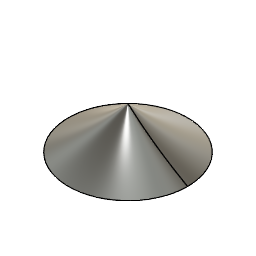
独自ミラー 試作品1 (Autodesk Fusion 360 design; units mm, degrees)
Autodesk Fusion 360 part; units mm, degrees
sketch "スケッチ2" plane through (0, 0, 0) normal (0, 0, 1) x (1, 0, 0)
  spline S0 degree 5 poles (25.9808, 45) (25.9662, 44.9918) (25.9371, 44.9754) (25.8935, 44.9508) (25.8354, 44.918) (25.7629, 44.8771) (25.6905, 44.8361) (25.6181, 44.7952) (25.5459, 44.7542) (25.4738, 44.7133) (25.4017, 44.6724) (25.3298, 44.6316) (25.2579, 44.5907) (25.1862, 44.5499) (25.1145, 44.509) (25.0429, 44.4682) (24.9715, 44.4274) (24.9001, 44.3866) (24.8288, 44.3459) (24.7576, 44.3051) (24.6865, 44.2644) (24.6155, 44.2236) (24.5446, 44.1829) (24.4738, 44.1422) (24.403, 44.1016) (24.3324, 44.0609) (24.2619, 44.0203) (24.1914, 43.9796) (24.1211, 43.939) (24.0508, 43.8984) (23.9806, 43.8578) (23.9106, 43.8172) (23.8406, 43.7767) (23.7707, 43.7361) (23.7009, 43.6956) (23.6312, 43.6551) (23.5616, 43.6146) (23.4921, 43.5741) (23.4227, 43.5336) (23.3533, 43.4932) (23.2841, 43.4528) (23.215, 43.4123) (23.1459, 43.3719) (23.0769, 43.3315) (23.0081, 43.2912) (22.9393, 43.2508) (22.8706, 43.2104) (22.802, 43.1701) (22.7335, 43.1298) (22.6651, 43.0895) (22.5968, 43.0492) (22.5286, 43.0089) (22.4604, 42.9687) (22.3924, 42.9284) (22.3244, 42.8882) (22.2566, 42.848) (22.1888, 42.8078) (22.1211, 42.7676) (22.0535, 42.7275) (21.986, 42.6873) (21.9186, 42.6472) (21.8513, 42.6071) (21.7841, 42.567) (21.717, 42.5269) (21.6499, 42.4868) (21.583, 42.4467) (21.5161, 42.4067) (21.4493, 42.3667) (21.3826, 42.3267) (21.316, 42.2867) (21.2495, 42.2467) (21.1831, 42.2067) (21.1168, 42.1668) (21.0506, 42.1268) (20.9844, 42.0869) (20.9184, 42.047) (20.8524, 42.0071) (20.7865, 41.9672) (20.7207, 41.9274) (20.655, 41.8875) (20.5894, 41.8477) (20.5239, 41.8079) (20.4585, 41.7681) (20.3931, 41.7283) (20.3279, 41.6885) (20.2627, 41.6488) (20.1976, 41.609) (20.1327, 41.5693) (20.0678, 41.5296) (20.0029, 41.4899) (19.9382, 41.4502) (19.8736, 41.4106) (19.809, 41.3709) (19.7446, 41.3313) (19.6802, 41.2917) (19.6159, 41.2521) (19.5517, 41.2125) (19.4876, 41.1729) (19.4236, 41.1334) (19.3597, 41.0938) (19.2959, 41.0543) (19.2321, 41.0148) (19.1684, 40.9753) (19.1049, 40.9358) (19.0414, 40.8963) (18.978, 40.8569) (18.9146, 40.8175) (18.8514, 40.778) (18.7883, 40.7386) (18.7252, 40.6993) (18.6622, 40.6599) (18.5993, 40.6205) (18.5365, 40.5812) (18.4738, 40.5419) (18.4112, 40.5025) (18.3487, 40.4632) (18.2862, 40.424) (18.2239, 40.3847) (18.1616, 40.3454) (18.0994, 40.3062) (18.0373, 40.267) (17.9753, 40.2278) (17.9133, 40.1886) (17.8515, 40.1494) (17.7897, 40.1103) (17.728, 40.0711) (17.6664, 40.032) (17.6049, 39.9929) (17.5435, 39.9538) (17.4822, 39.9147) (17.4209, 39.8756) (17.3597, 39.8366) (17.2987, 39.7976) (17.2377, 39.7585) (17.1768, 39.7195) (17.1159, 39.6805) (17.0552, 39.6416) (16.9945, 39.6026) (16.934, 39.5637) (16.8735, 39.5247) (16.8131, 39.4858) (16.7527, 39.4469) (16.6925, 39.408) (16.6324, 39.3692) (16.5723, 39.3303) (16.5123, 39.2915) (16.4524, 39.2527) (16.3926, 39.2139) (16.3329, 39.1751) (16.2732, 39.1363) (16.2136, 39.0975) (16.1542, 39.0588) (16.0948, 39.0201) (16.0355, 38.9814) (15.9762, 38.9427) (15.9171, 38.904) (15.858, 38.8653) (15.799, 38.8267) (15.7401, 38.788) (15.6813, 38.7494) (15.6226, 38.7108) (15.5639, 38.6722) (15.5054, 38.6336) (15.4469, 38.5951) (15.3885, 38.5565) (15.3302, 38.518) (15.2719, 38.4795) (15.2138, 38.441) (15.1557, 38.4025) (15.0977, 38.3641) (15.0398, 38.3256) (14.982, 38.2872) (14.9242, 38.2488) (14.8666, 38.2104) (14.809, 38.172) (14.7515, 38.1336) (14.6941, 38.0952) (14.6367, 38.0569) (14.5795, 38.0186) (14.5223, 37.9803) (14.4652, 37.942) (14.4082, 37.9037) (14.3513, 37.8654) (14.2944, 37.8272) (14.2377, 37.7889) (14.181, 37.7507) (14.1244, 37.7125) (14.0679, 37.6743) (14.0114, 37.6362) (13.955, 37.598) (13.8988, 37.5599) (13.8426, 37.5217) (13.7864, 37.4836) (13.7304, 37.4455) (13.6744, 37.4075) (13.6186, 37.3694) (13.5628, 37.3314) (13.507, 37.2933) (13.4514, 37.2553) (13.3958, 37.2173) (13.3403, 37.1793) (13.2849, 37.1414) (13.2296, 37.1034) (13.1744, 37.0655) (13.1192, 37.0276) (13.0641, 36.9897) (13.0091, 36.9518) (12.9542, 36.9139) (12.8994, 36.876) (12.8446, 36.8382) (12.7899, 36.8004) (12.7353, 36.7626) (12.6808, 36.7248) (12.6263, 36.687) (12.5719, 36.6492) (12.5176, 36.6115) (12.4634, 36.5737) (12.4093, 36.536) (12.3552, 36.4983) (12.3012, 36.4606) (12.2473, 36.423) (12.1935, 36.3853) (12.1398, 36.3477) (12.0861, 36.31) (12.0325, 36.2724) (11.979, 36.2349) (11.9256, 36.1973) (11.8722, 36.1597) (11.8189, 36.1222) (11.7657, 36.0846) (11.7126, 36.0471) (11.6595, 36.0096) (11.6066, 35.9722) (11.5537, 35.9347) (11.5009, 35.8972) (11.4481, 35.8598) (11.3955, 35.8224) (11.3429, 35.785) (11.2904, 35.7476) (11.2379, 35.7102) (11.1856, 35.6729) (11.1333, 35.6356) (11.0811, 35.5982) (11.029, 35.5609) (10.9769, 35.5236) (10.925, 35.4864) (10.8731, 35.4491) (10.8212, 35.4119) (10.7695, 35.3746) (10.7178, 35.3374) (10.6662, 35.3002) (10.6147, 35.2631) (10.5633, 35.2259) (10.5119, 35.1888) (10.4606, 35.1516) (10.4094, 35.1145) (10.3583, 35.0774) (10.3072, 35.0403) (10.2562, 35.0033) (10.2053, 34.9662) (10.1545, 34.9292) (10.1037, 34.8922) (10.053, 34.8552) (10.0024, 34.8182) (9.9519, 34.7812) (9.9014, 34.7443) (9.851, 34.7073) (9.8007, 34.6704) (9.7505, 34.6335) (9.7003, 34.5966) (9.6502, 34.5597) (9.6002, 34.5229) (9.5502, 34.4861) (9.5004, 34.4492) (9.4506, 34.4124) (9.4009, 34.3756) (9.3512, 34.3389) (9.3016, 34.3021) (9.2521, 34.2654) (9.2027, 34.2286) (9.1534, 34.1919) (9.1041, 34.1552) (9.0549, 34.1186) (9.0057, 34.0819) (8.9567, 34.0453) (8.9077, 34.0086) (8.8588, 33.972) (8.8099, 33.9354) (8.7612, 33.8989) (8.7125, 33.8623) (8.6639, 33.8258) (8.6153, 33.7892) (8.5668, 33.7527) (8.5184, 33.7162) (8.4701, 33.6797) (8.4218, 33.6433) (8.3737, 33.6068) (8.3255, 33.5704) (8.2775, 33.534) (8.2295, 33.4976) (8.1816, 33.4612) (8.1338, 33.4249) (8.0861, 33.3885) (8.0384, 33.3522) (7.9908, 33.3159) (7.9432, 33.2796) (7.8958, 33.2433) (7.8484, 33.2071) (7.801, 33.1708) (7.7538, 33.1346) (7.7066, 33.0984) (7.6595, 33.0622) (7.6124, 33.026) (7.5655, 32.9899) (7.5186, 32.9537) (7.4717, 32.9176) (7.425, 32.8815) (7.3783, 32.8454) (7.3317, 32.8093) (7.2851, 32.7733) (7.2387, 32.7372) (7.1923, 32.7012) (7.1459, 32.6652) (7.0997, 32.6292) (7.0535, 32.5933) (7.0073, 32.5573) (6.9613, 32.5214) (6.9153, 32.4855) (6.8694, 32.4496) (6.8235, 32.4137) (6.7778, 32.3778) (6.7321, 32.342) (6.6864, 32.3061) (6.6408, 32.2703) (6.5953, 32.2345) (6.5499, 32.1988) (6.5046, 32.163) (6.4593, 32.1273) (6.414, 32.0915) (6.3689, 32.0558) (6.3238, 32.0201) (6.2788, 31.9845) (6.2338, 31.9488) (6.189, 31.9132) (6.1441, 31.8776) (6.0994, 31.842) (6.0547, 31.8064) (6.0101, 31.7708) (5.9656, 31.7353) (5.9211, 31.6998) (5.8767, 31.6643) (5.8324, 31.6288) (5.7881, 31.5933) (5.7439, 31.5579) (5.6998, 31.5224) (5.6557, 31.487) (5.6117, 31.4516) (5.5678, 31.4163) (5.5239, 31.3809) (5.4801, 31.3456) (5.4364, 31.3103) (5.3927, 31.275) (5.3491, 31.2397) (5.3056, 31.2044) (5.2621, 31.1692) (5.2187, 31.1339) (5.1754, 31.0987) (5.1321, 31.0636) (5.0889, 31.0284) (5.0458, 30.9933) (5.0027, 30.9581) (4.9597, 30.923) (4.9168, 30.8879) (4.8739, 30.8529) (4.8311, 30.8178) (4.7884, 30.7828) (4.7457, 30.7478) (4.7031, 30.7128) (4.6606, 30.6778) (4.6181, 30.6429) (4.5757, 30.608) (4.5333, 30.5731) (4.491, 30.5382) (4.4488, 30.5033) (4.4067, 30.4685) (4.3646, 30.4337) (4.3226, 30.3989) (4.2806, 30.3641) (4.2387, 30.3293) (4.1969, 30.2946) (4.1551, 30.2599) (4.1134, 30.2252) (4.0718, 30.1905) (4.0302, 30.1559) (3.9887, 30.1213) (3.9472, 30.0867) (3.9058, 30.0521) (3.8645, 30.0175) (3.8232, 29.983) (3.782, 29.9485) (3.7409, 29.914) (3.6998, 29.8795) (3.6588, 29.8451) (3.6179, 29.8107) (3.577, 29.7763) (3.5362, 29.7419) (3.4954, 29.7076) (3.4547, 29.6732) (3.4141, 29.6389) (3.3735, 29.6047) (3.333, 29.5704) (3.2925, 29.5362) (3.2521, 29.502) (3.2118, 29.4678) (3.1715, 29.4337) (3.1313, 29.3996) (3.0912, 29.3655) (3.0511, 29.3314) (3.011, 29.2974) (2.9711, 29.2634) (2.9311, 29.2294) (2.8913, 29.1955) (2.8515, 29.1615) (2.8118, 29.1276) (2.7721, 29.0938) (2.7325, 29.0599) (2.6929, 29.0261) (2.6534, 28.9924) (2.614, 28.9586) (2.5746, 28.9249) (2.5353, 28.8912) (2.496, 28.8576) (2.4568, 28.824) (2.4177, 28.7904) (2.3786, 28.7568) (2.3395, 28.7233) (2.3006, 28.6898) (2.2616, 28.6564) (2.2228, 28.623) (2.1839, 28.5896) (2.1452, 28.5563) (2.1065, 28.523) (2.0678, 28.4897) (2.0292, 28.4565) (1.9907, 28.4234) (1.9522, 28.3902) (1.9138, 28.3571) (1.8754, 28.3241) (1.8371, 28.2911) (1.7988, 28.2581) (1.7606, 28.2252) (1.7224, 28.1924) (1.6843, 28.1596) (1.6462, 28.1268) (1.6082, 28.0941) (1.5702, 28.0615) (1.5323, 28.0289) (1.4944, 27.9963) (1.4566, 27.9639) (1.4188, 27.9314) (1.3811, 27.8991) (1.3434, 27.8668) (1.3058, 27.8346) (1.2682, 27.8024) (1.2306, 27.7704) (1.1931, 27.7384) (1.1556, 27.7064) (1.1182, 27.6746) (1.0808, 27.6428) (1.0434, 27.6112) (1.0061, 27.5796) (0.9688, 27.5481) (0.9316, 27.5168) (0.8944, 27.4855) (0.8572, 27.4544) (0.82, 27.4234) (0.7829, 27.3925) (0.7457, 27.3618) (0.7087, 27.3312) (0.6716, 27.3007) (0.6345, 27.2705) (0.5975, 27.2404) (0.5604, 27.2105) (0.5234, 27.1808) (0.4863, 27.1514) (0.4493, 27.1222) (0.4122, 27.0933) (0.3751, 27.0647) (0.338, 27.0364) (0.3008, 27.0085) (0.2636, 26.981) (0.2264, 26.9539) (0.189, 26.9275) (0.1515, 26.9017) (0.1139, 26.8767) (0.0761, 26.8527) (0.0458, 26.8342) (0.0229, 26.8207) (0.0076, 26.8119) (0, 26.8076) knots 0 0 0 0 0 0 0.0020202 0.0040404 0.00606061 0.00808081 0.01010101 0.01212121 0.01414141 0.01616162 0.01818182 0.02020202 0.02222222 0.02424242 0.02626263 0.02828283 0.03030303 0.03232323 0.03434343 0.03636364 0.03838384 0.04040404 0.04242424 0.04444444 0.04646465 0.04848485 0.05050505 0.05252525 0.05454545 0.05656566 0.05858586 0.06060606 0.06262626 0.06464646 0.06666667 0.06868687 0.07070707 0.07272727 0.07474747 0.07676768 0.07878788 0.08080808 0.08282828 0.08484848 0.08686869 0.08888889 0.09090909 0.09292929 0.09494949 0.0969697 0.0989899 0.1010101 0.1030303 0.10505051 0.10707071 0.10909091 0.11111111 0.11313131 0.11515152 0.11717172 0.11919192 0.12121212 0.12323232 0.12525253 0.12727273 0.12929293 0.13131313 0.13333333 0.13535354 0.13737374 0.13939394 0.14141414 0.14343434 0.14545455 0.14747475 0.14949495 0.15151515 0.15353535 0.15555556 0.15757576 0.15959596 0.16161616 0.16363636 0.16565657 0.16767677 0.16969697 0.17171717 0.17373737 0.17575758 0.17777778 0.17979798 0.18181818 0.18383838 0.18585859 0.18787879 0.18989899 0.19191919 0.19393939 0.1959596 0.1979798 0.2 0.2020202 0.2040404 0.20606061 0.20808081 0.21010101 0.21212121 0.21414141 0.21616162 0.21818182 0.22020202 0.22222222 0.22424242 0.22626263 0.22828283 0.23030303 0.23232323 0.23434343 0.23636364 0.23838384 0.24040404 0.24242424 0.24444444 0.24646465 0.24848485 0.25050505 0.25252525 0.25454545 0.25656566 0.25858586 0.26060606 0.26262626 0.26464646 0.26666667 0.26868687 0.27070707 0.27272727 0.27474747 0.27676768 0.27878788 0.28080808 0.28282828 0.28484848 0.28686869 0.28888889 0.29090909 0.29292929 0.29494949 0.2969697 0.2989899 0.3010101 0.3030303 0.30505051 0.30707071 0.30909091 0.31111111 0.31313131 0.31515152 0.31717172 0.31919192 0.32121212 0.32323232 0.32525253 0.32727273 0.32929293 0.33131313 0.33333333 0.33535354 0.33737374 0.33939394 0.34141414 0.34343434 0.34545455 0.34747475 0.34949495 0.35151515 0.35353535 0.35555556 0.35757576 0.35959596 0.36161616 0.36363636 0.36565657 0.36767677 0.36969697 0.37171717 0.37373737 0.37575758 0.37777778 0.37979798 0.38181818 0.38383838 0.38585859 0.38787879 0.38989899 0.39191919 0.39393939 0.3959596 0.3979798 0.4 0.4020202 0.4040404 0.40606061 0.40808081 0.41010101 0.41212121 0.41414141 0.41616162 0.41818182 0.42020202 0.42222222 0.42424242 0.42626263 0.42828283 0.43030303 0.43232323 0.43434343 0.43636364 0.43838384 0.44040404 0.44242424 0.44444444 0.44646465 0.44848485 0.45050505 0.45252525 0.45454545 0.45656566 0.45858586 0.46060606 0.46262626 0.46464646 0.46666667 0.46868687 0.47070707 0.47272727 0.47474747 0.47676768 0.47878788 0.48080808 0.48282828 0.48484848 0.48686869 0.48888889 0.49090909 0.49292929 0.49494949 0.4969697 0.4989899 0.5010101 0.5030303 0.50505051 0.50707071 0.50909091 0.51111111 0.51313131 0.51515152 0.51717172 0.51919192 0.52121212 0.52323232 0.52525253 0.52727273 0.52929293 0.53131313 0.53333333 0.53535354 0.53737374 0.53939394 0.54141414 0.54343434 0.54545455 0.54747475 0.54949495 0.55151515 0.55353535 0.55555556 0.55757576 0.55959596 0.56161616 0.56363636 0.56565657 0.56767677 0.56969697 0.57171717 0.57373737 0.57575758 0.57777778 0.57979798 0.58181818 0.58383838 0.58585859 0.58787879 0.58989899 0.59191919 0.59393939 0.5959596 0.5979798 0.6 0.6020202 0.6040404 0.60606061 0.60808081 0.61010101 0.61212121 0.61414141 0.61616162 0.61818182 0.62020202 0.62222222 0.62424242 0.62626263 0.62828283 0.63030303 0.63232323 0.63434343 0.63636364 0.63838384 0.64040404 0.64242424 0.64444444 0.64646465 0.64848485 0.65050505 0.65252525 0.65454545 0.65656566 0.65858586 0.66060606 0.66262626 0.66464646 0.66666667 0.66868687 0.67070707 0.67272727 0.67474747 0.67676768 0.67878788 0.68080808 0.68282828 0.68484848 0.68686869 0.68888889 0.69090909 0.69292929 0.69494949 0.6969697 0.6989899 0.7010101 0.7030303 0.70505051 0.70707071 0.70909091 0.71111111 0.71313131 0.71515152 0.71717172 0.71919192 0.72121212 0.72323232 0.72525253 0.72727273 0.72929293 0.73131313 0.73333333 0.73535354 0.73737374 0.73939394 0.74141414 0.74343434 0.74545455 0.74747475 0.74949495 0.75151515 0.75353535 0.75555556 0.75757576 0.75959596 0.76161616 0.76363636 0.76565657 0.76767677 0.76969697 0.77171717 0.77373737 0.77575758 0.77777778 0.77979798 0.78181818 0.78383838 0.78585859 0.78787879 0.78989899 0.79191919 0.79393939 0.7959596 0.7979798 0.8 0.8020202 0.8040404 0.80606061 0.80808081 0.81010101 0.81212121 0.81414141 0.81616162 0.81818182 0.82020202 0.82222222 0.82424242 0.82626263 0.82828283 0.83030303 0.83232323 0.83434343 0.83636364 0.83838384 0.84040404 0.84242424 0.84444444 0.84646465 0.84848485 0.85050505 0.85252525 0.85454545 0.85656566 0.85858586 0.86060606 0.86262626 0.86464646 0.86666667 0.86868687 0.87070707 0.87272727 0.87474747 0.87676768 0.87878788 0.88080808 0.88282828 0.88484848 0.88686869 0.88888889 0.89090909 0.89292929 0.89494949 0.8969697 0.8989899 0.9010101 0.9030303 0.90505051 0.90707071 0.90909091 0.91111111 0.91313131 0.91515152 0.91717172 0.91919192 0.92121212 0.92323232 0.92525253 0.92727273 0.92929293 0.93131313 0.93333333 0.93535354 0.93737374 0.93939394 0.94141414 0.94343434 0.94545455 0.94747475 0.94949495 0.95151515 0.95353535 0.95555556 0.95757576 0.95959596 0.96161616 0.96363636 0.96565657 0.96767677 0.96969697 0.97171717 0.97373737 0.97575758 0.97777778 0.97979798 0.98181818 0.98383838 0.98585859 0.98787879 0.98989899 0.99191919 0.99393939 0.9959596 0.9979798 1 1 1 1 1 1
  line L0 (25.9808, 45) -> (0, 45)
  line L1 (0, 45) -> (0, 26.8076)
  point P0 (25.5139, 44.7361)
  point P1 (25.0539, 44.4745)
  point P2 (24.6006, 44.2151)
  point P3 (24.154, 43.958)
  point P4 (23.7139, 43.7031)
  point P5 (23.2802, 43.4505)
  point P6 (22.8527, 43.1999)
  point P7 (22.4314, 42.9515)
  point P8 (22.016, 42.7052)
  point P9 (21.6066, 42.4609)
  point P10 (21.203, 42.2187)
  point P11 (20.8051, 41.9785)
  point P12 (20.4128, 41.7402)
  point P13 (20.0259, 41.504)
  point P14 (19.6444, 41.2696)
  point P15 (19.2682, 41.0372)
  point P16 (18.8972, 40.8066)
  point P17 (18.5313, 40.5779)
  point P18 (18.1704, 40.351)
  point P19 (17.8144, 40.1259)
  point P20 (17.4632, 39.9026)
  point P21 (17.1167, 39.681)
  point P22 (16.7749, 39.4612)
  point P23 (16.4377, 39.2431)
  point P24 (16.105, 39.0267)
  point P25 (15.7767, 38.812)
  point P26 (15.4527, 38.5989)
  point P27 (15.1329, 38.3874)
  point P28 (14.8174, 38.1776)
  point P29 (14.506, 37.9693)
  point P30 (14.1986, 37.7626)
  point P31 (13.8952, 37.5574)
  point P32 (13.5957, 37.3538)
  point P33 (13.3, 37.1517)
  point P34 (13.0081, 36.9511)
  point P35 (12.72, 36.7519)
  point P36 (12.4355, 36.5542)
  point P37 (12.1545, 36.358)
  point P38 (11.8771, 36.1632)
  point P39 (11.6032, 35.9698)
  point P40 (11.3327, 35.7777)
  point P41 (11.0656, 35.5871)
  point P42 (10.8017, 35.3978)
  point P43 (10.5411, 35.2099)
  point P44 (10.2838, 35.0233)
  point P45 (10.0295, 34.838)
  point P46 (9.7784, 34.654)
  point P47 (9.5303, 34.4713)
  point P48 (9.2852, 34.2899)
  point P49 (9.0431, 34.1098)
  point P50 (8.8038, 33.9309)
  point P51 (8.5675, 33.7532)
  point P52 (8.3339, 33.5767)
  point P53 (8.1031, 33.4015)
  point P54 (7.8751, 33.2275)
  point P55 (7.6497, 33.0547)
  point P56 (7.427, 32.883)
  point P57 (7.2068, 32.7125)
  point P58 (6.9893, 32.5432)
  point P59 (6.7742, 32.375)
  point P60 (6.5617, 32.208)
  point P61 (6.3516, 32.0421)
  point P62 (6.1439, 31.8773)
  point P63 (5.9385, 31.7137)
  point P64 (5.7355, 31.5512)
  point P65 (5.5349, 31.3897)
  point P66 (5.3364, 31.2294)
  point P67 (5.1403, 31.0702)
  point P68 (4.9463, 30.912)
  point P69 (4.7545, 30.755)
  point P70 (4.5648, 30.599)
  point P71 (4.3772, 30.4441)
  point P72 (4.1917, 30.2903)
  point P73 (4.0082, 30.1376)
  point P74 (3.8268, 29.9859)
  point P75 (3.6473, 29.8354)
  point P76 (3.4698, 29.686)
  point P77 (3.2942, 29.5376)
  point P78 (3.1205, 29.3904)
  point P79 (2.9487, 29.2443)
  point P80 (2.7787, 29.0994)
  point P81 (2.6105, 28.9556)
  point P82 (2.4441, 28.813)
  point P83 (2.2794, 28.6717)
  point P84 (2.1165, 28.5316)
  point P85 (1.9552, 28.3928)
  point P86 (1.7957, 28.2555)
  point P87 (1.6378, 28.1196)
  point P88 (1.4815, 27.9852)
  point P89 (1.3268, 27.8526)
  point P90 (1.1736, 27.7218)
  point P91 (1.022, 27.5931)
  point P92 (0.8719, 27.4667)
  point P93 (0.7232, 27.3432)
  point P94 (0.576, 27.2231)
  point P95 (0.4301, 27.1073)
  point P96 (0.2856, 26.9973)
  point P97 (0.1422, 26.8957)
  constraint horizontal L0
  constraint perpendicular L0 L1
revolve "回転1" add sketch "スケッチ2" angle 360 about axis through (0, 45, 0) along (0, -1, 0)
move_body "移動1" bodies 1 to x (1, 0, 0) y (0, 0, -1) z (0, 1, 0) at (0, 45, 45)
move_body "移動2" bodies 1 to x (1, 0, 0) y (0, 1, 0) z (0, 0, 1) at (0, -45, 0)
